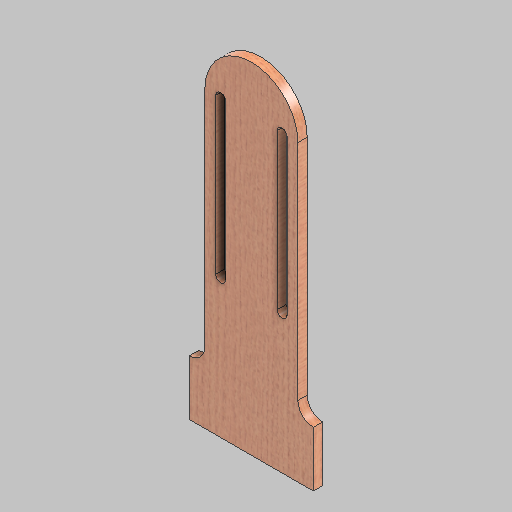
# Autodesk Inventor part: Painel Vertical
Saved by Autodesk Inventor 2025.2 (Build 292293000, 293)
## iProperties
Created: 2024-04-26
Part Number: Painel Vertical
Material: Genérico
Document SubType Name: Modeling
Designer: phmca
Density: 1 g/cm^3
Appearance: Padrão
Author: phmca
Autodesk Inventor part; units mm, degrees
ref_plane "YZ Plane" through (0, 0, 0) normal (1, 0, 0) x (0, 1, 0)
ref_plane "XZ Plane" through (0, 0, 0) normal (0, 1, 0) x (-1, 0, 0)
ref_plane "XY Plane" through (0, 0, 0) normal (0, 0, 1) x (1, 0, 0)
sketch "Esboço1" plane through (0, 0, 0) normal (0, 1, 0) x (-1, 0, 0)
  line L0 (-100, 7.5) -> (100, 7.5)
  line L1 (100, 7.5) -> (100, -7.5)
  line L2 (100, -7.5) -> (-100, -7.5)
  line L3 (-100, -7.5) -> (-100, 7.5)
  line L4 (-100, 7.5) -> (100, -7.5) construction
  line L5 (100, 7.5) -> (-100, -7.5) construction
  point P0 (0, 0)
  dimension "d0" = 200
  dimension "d1" = 15
  constraints: 12 end point, 2 midpoint, 2 parallel, 1 horizontal, 1 perpendicular
  measures "d0" distance of L1.end L2.end
  measures "d1" distance of L0.end L1.end
extrude "Extrusão1" add sketch "Esboço1" along normal mid plane 600
sketch "Esboço2" plane through (-100, 300, 7.5) normal (0, 0, 1) x (1, 0, 0)
  line L0 (0, 0) -> (200, 0) projected
  line L1 (100, 0) -> (100, 69.4125)
  line L2 (100, -51) -> (100, -126) construction
  line L3 (-27.4688, -551) -> (246.7453, -551) construction
  line L4 (200, -600) -> (0, -600) projected
  line L5 (25, -126) -> (25, -486)
  line L6 (175, -126) -> (175, -486)
  arc A0 (175, -126) -> (25, -126) centre (100, -126) ccw
  line L7 (200, -600) -> (200, 0) projected
  line L8 (0, -600) -> (0, 0) projected
  line L9 (0, -511) -> (25, -511) construction
  line L10 (175, -511) -> (200, -511) construction
  arc A1 (0, -511) -> (25, -486) centre (0, -486) ccw
  line L11 (25, -486) -> (25, -511) construction
  arc A2 (175, -486) -> (200, -511) centre (200, -486) ccw
  line L12 (175, -486) -> (175, -511) construction
  point P0 (100, -300)
  dimension "d7" = 49
  dimension "d9" = 150
  dimension "d10" = 500
  dimension "d11" = 40
  constraints: 18 end point, 10 tangent, 8 perpendicular, 7 point on circle, 4 point on line, 3 centre point, 2 collinear, 2 horizontal, 2 vertical, 1 coincident, 1 midpoint
  measures "d7" distance between parallel lines of L3 L4
  measures "d9" distance between parallel lines of L6 L5
  measures "d10" distance from line of L3 point (100, -51)
  measures "d11" distance between parallel lines of L3 L9
extrude "Extrusão2" cut sketch "Esboço2" against normal up to surface (15 mm away) contours L0 L7 A2 L6 A0 L5 A1 L8
extrude "Extrusão3" add sketch "Esboço2" against normal up to surface (15 mm away) separate body contours L0 L7 A2 L6 A0 L5 A1 L8
sketch "Esboço3" plane through (100, -300, -7.5) normal (0, 0, -1) x (-1, 0, 0)
  arc A0 (58.5, 474) -> (42.5, 474) centre (50.5, 474) ccw
  arc A1 (157.5, 474) -> (141.5, 474) centre (149.5, 474) ccw
  line L0 (50.5, 474) -> (149.5, 474) construction
  arc A2 (175, 474) -> (25, 474) centre (100, 474) ccw projected
  line L1 (100, 474) -> (100, 578.5604) construction
  line L2 (100, 474) -> (100, 224) construction
  arc A3 (42.5, 224) -> (58.5, 224) centre (50.5, 224) ccw
  arc A4 (141.5, 224) -> (157.5, 224) centre (149.5, 224) ccw
  line L3 (50.5, 224) -> (149.5, 224) construction
  line L4 (42.5, 474) -> (42.5, 224)
  line L5 (58.5, 224) -> (58.5, 474)
  line L6 (141.5, 474) -> (141.5, 224)
  line L7 (157.5, 224) -> (157.5, 474)
  point P0 (100, 300)
  dimension "d16" = 16
  dimension "d17" = 16
  dimension "d18" = 99
  dimension "d19" = 16
  dimension "d20" = 16
  dimension "d21" = 99
  dimension "d22" = 250
  constraints: 16 end point, 8 point on circle, 4 centre point, 4 point on line, 4 tangent, 3 midpoint, 2 horizontal, 2 vertical, 1 collinear
  measures "d16" diameter of A0
  measures "d17" diameter of A1
  measures "d18" distance of L0.start L0.end
  measures "d19" diameter of A3
  measures "d20" diameter of A4
  measures "d21" distance of L3.start L3.end
  measures "d22" distance between parallel lines of L3 L0
extrude "Extrusão4" cut sketch "Esboço3" against normal up to surface (15 mm away)
sketch "Esboço4" plane through (-100, -300, 7.5) normal (0, 0, 1) x (1, 0, 0)
  arc A0 (141.5, 224) -> (157.5, 224) centre (149.5, 224) ccw projected
  arc A1 (157.5, 474) -> (141.5, 474) centre (149.5, 474) ccw projected
  line L0 (149.5, 224) -> (149.5, 474) construction
  line L1 (149.5, 349) -> (241.6244, 349) construction
  point P0 (100, 300)
  constraints: 4 end point, 1 horizontal, 1 midpoint, 1 vertical
